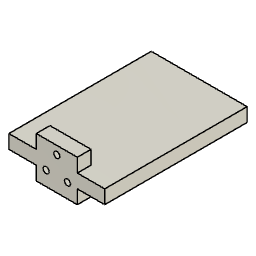
gurigri_plate (Autodesk Fusion 360 design; units mm, degrees)
Autodesk Fusion 360 part; units mm, degrees
box "直方体プリミティブ1" add length 40 width 35 height 5 placed x (0, 1, 0) y (-1, 0, 0) z (0, 0, 1) at (35, 0, 0) makes body 1
sketch "スケッチ2" plane through (0, 0, 5) normal (0, 0, 1) x (-1, 0, 0)
  line L0 (-35, -40) -> (0, -40)
  line L1 (0, -40) -> (0, 0)
  line L2 (0, 0) -> (-35, 0)
  line L3 (-35, 0) -> (-35, -40)
sketch "スケッチ3" plane through (0, 0, 5) normal (0, 0, 1) x (-1, 0, 0)
  line L0 (0, 0) -> (-35, -40)
  line L1 (-35, -40) -> (-35, 0)
  line L2 (-35, 0) -> (0, -40)
  constraint coincident L0.start origin
  constraint vertical L1
sketch "スケッチ4" plane through (0, 0, 5) normal (0, 0, 1) x (-1, 0, 0)
  line L0 (-17.5, -20) -> (-17.5, 0)
  line L1 (-17.5, 0) -> (-17.5, -5)
  constraint vertical L0
  constraint coincident L0 L1.end
sketch "スケッチ5" plane through (0, 0, 5) normal (0, 0, 1) x (-1, 0, 0)
  line L0 (-17.5, -5) -> (-25, -5)
  line L1 (-25, -5) -> (-10, -5)
  line L2 (-10, -5) -> (-10, 0)
  line L3 (-10, 0) -> (-25, 0)
  line L4 (-25, 0) -> (-25, -5)
  constraint horizontal L0
  constraint parallel L0 L1
  constraint perpendicular L1 L2
  constraint perpendicular L2 L3
  constraint perpendicular L1 L4
box "直方体プリミティブ2" add length 5 width 15 height 15 placed x (0, -1, 0) y (1, 0, 0) z (0, 0, 1) at (10, 5, 5) bodies 1
sketch "スケッチ7" plane through (0, 5, 0) normal (0, 1, 0) x (-1, 0, 0)
  line L0 (-25, 20) -> (-25, 5)
  line L1 (-25, 5) -> (-10, 5)
  line L2 (-10, 5) -> (-10, 20)
  line L3 (-10, 20) -> (-25, 20)
  line L4 (-25, 20) -> (-10, 5)
  line L5 (-10, 20) -> (-25, 5)
  constraint coincident L0.start L3.end
  constraint coincident L1.end L2.start
  constraint coincident L2.end L3.start
  constraint coincident L0.end L1.start
sketch "スケッチ8" plane through (0, 5, 0) normal (0, 1, 0) x (-1, 0, 0)
  circle A0 centre (-17.5, 12.5) radius 4.5
  line L0 (-17.5, 17) -> (-21.3971, 10.25)
  line L1 (-21.3971, 10.25) -> (-13.6029, 10.25)
  line L2 (-13.6029, 10.25) -> (-17.5, 17)
  point P0 (-17.5, 12.5)
  dimension "d11" = 9
  constraint coincident P0 A0.centre
  constraint coincident A0 L0.start
  measures "d11" diameter of A0
hole "穴1" at (13.6029, 5, 10.25) direction (0, -1, 0) diameter 2.2 depth 5 tip angle 180 bodies 1
hole "穴2" at (21.3971, 5, 10.25) direction (0, -1, 0) diameter 2.2 depth 5 tip angle 180 bodies 1
hole "穴3" at (17.5, 5, 17) direction (0, -1, 0) diameter 2.2 depth 5 tip angle 180 bodies 1
split "分割1" by plane through (35, 0, 5) normal (0, 0, 1) bodies 1 makes body 2 at (13.2354, 0, 16.0188)
move_body "移動1" bodies 1 to x (1, 0, 0) y (0, 1, 0) z (0, 0, 1) at (0, 0, 10)
copy_body "ボディのコピーと貼り付け1" bodies 2 makes body 3
delete_face "面を削除1" 1 faces at (13.6577, 3.3333, 11.3486) on bodies 3
delete_face "面を削除2" 1 faces at (21.5066, 3.3333, 9.1555) on bodies 3
delete_face "面を削除3" 1 faces at (18.2071, 3.3333, 16.1574) on bodies 3
copy_body "ボディのコピーと貼り付け2" bodies 1 makes body 4
combine "結合1" operation cut target body 4 tool bodies 3
move_face "面をオフセット1" offset 12 1 faces at (23.3333, 40, 11.6667) on bodies 4
sketch "スケッチ9" plane through (0, 5, 0) normal (0, 1, 0) x (-1, 0, 0)
sketch "スケッチ10" plane through (0, 0, 0) normal (0, 1, 0) x (1, 0, 0)
sketch "スケッチ11" plane through (0, 0, 0) normal (0, 1, 0) x (1, 0, 0)
sketch "スケッチ12" plane through (0, 5, 0) normal (0, 1, 0) x (-1, 0, 0)
sketch "スケッチ13" plane through (0, 0, 0) normal (0, 1, 0) x (1, 0, 0)
cylinder "円柱プリミティブ1" add diameter 4 height 10 placed x (1, 0, 0) y (0, 0, -1) z (0, 1, 0) at (21.3972, 5, 10.25) separate body makes body 5
cylinder "円柱プリミティブ2" add diameter 4 height 10 placed x (1, 0, 0) y (0, 0, -1) z (0, 1, 0) at (13.603, 5, 10.25) separate body makes body 6
combine "結合2" operation cut target body 4 tool bodies 5 6
chamfer "面取り1" distance 2 angle 45 1 edges at (21.3972, 15, 10) on bodies 4
chamfer "面取り2" distance 2 angle 45 1 edges at (13.603, 15, 10) on bodies 4
cylinder "円柱プリミティブ3" add diameter 4 height 10 placed x (1, 0, 0) y (0, 0, -1) z (0, 1, 0) at (17.5, 0, 17) separate body makes body 7
move_body "移動2" bodies 7 to x (1, 0, 0) y (0, 1, 0) z (0, 0, 1) at (0, 5, 0)
combine "結合3" operation cut target body 4 tool bodies 7
combine "結合4" operation add target body 4 tool bodies 2
delete_body "RemoveBody2" bodies 1
